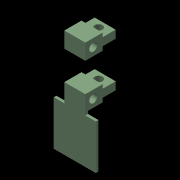
# Autodesk Inventor part: Bearing1
Saved by Autodesk Inventor 2020 (Build 240168000, 168)
## iProperties
Created: 2019-08-05
Part Number: Bearing1
Document SubType Name: Modeling
Designer: Administrator
Density: 1 g/cm^3
Mass: 0.988579 g
Surface Area: 15.6045 cm^2
Volume: 0.988579 cm^3
Material: 一般
Appearance: Green Pastel
Author: Administrator
Autodesk Inventor part; units mm, degrees
ref_plane "YZ Plane" through (0, 0, 0) normal (1, 0, 0) x (0, 1, 0)
ref_plane "XZ Plane" through (0, 0, 0) normal (0, 1, 0) x (-1, 0, 0)
ref_plane "XY Plane" through (0, 0, 0) normal (0, 0, 1) x (1, 0, 0)
sketch "Sketch1" plane through (0, 0, 0) normal (0, 0, 1) x (1, 0, 0)
  circle A0 centre (0, 0) radius 1.5
  line L0 (2.5, 2.5) -> (2.5, -2.5)
  line L1 (2.5, -2.5) -> (-2.5, -2.5)
  line L2 (-2.5, -2.5) -> (-2.5, 2.5)
  line L3 (-2.5, 2.5) -> (2.5, 2.5)
  dimension "d0" = 3
  dimension "d1" = 5
  constraints: 8 end point, 1 centre point, 1 coincident, 10 other
  measures "d0" diameter of A0
  measures "d1" distance of L2.end L0.start
extrude "Extrusion1" add sketch "Sketch1" along normal blind 3
pattern_linear "Rectangular Pattern1" count 2 spacing 17 along (0, 0, 1) of "Extrusion1"
sketch "Sketch2" plane through (0, 0, 0) normal (1, 0, 0) x (0, 1, 0)
  line L0 (-2.5, 17) -> (-2.5, 20) projected
  line L1 (-2.5, 0) -> (-2.5, 3) projected
  line L2 (-2.5, 18.5) -> (-6.05, 18.5) construction
  line L3 (-6.05, 18.5) -> (-6.05, 1.5) construction
  line L4 (-6.05, 1.5) -> (-2.5, 1.5) construction
  line L5 (2.5, 3) -> (-2.5, 3) projected
  line L6 (2.5, 17) -> (-2.5, 17) projected
  line L7 (0, 16.4638) -> (0, 3) construction
  circle A0 centre (-6.05, 18.5) radius 1.5
  circle A1 centre (-6.05, 1.5) radius 1.5
  line L8 (-2.5, 20) -> (-2.5, 21.5)
  line L9 (-2.5, 21.5) -> (-9.05, 21.5)
  line L10 (-9.05, 21.5) -> (-9.05, 15.5)
  line L11 (-9.05, 15.5) -> (-2.5, 15.5)
  line L12 (-2.5, 15.5) -> (-2.5, 17)
  line L13 (-6.05, 10) -> (0, 10) construction
  line L14 (-2.5, 3) -> (-2.5, 0)
  line L15 (-2.5, 1.5) -> (-6.05, 1.5) construction
  circle A2 centre (-6.05, 1.5) radius 1.5
  line L16 (-2.5, 0) -> (-2.5, -1.5)
  line L17 (-2.5, -1.5) -> (-9.05, -1.5)
  line L18 (-9.05, -1.5) -> (-9.05, 4.5)
  line L19 (-9.05, 4.5) -> (-2.5, 4.5)
  line L20 (-2.5, 4.5) -> (-2.5, 3)
  line L21 (-2.5, 17) -> (-2.5, 20)
  dimension "d7" = 6.05
  dimension "d8" = 3
  dimension "d9" = 3
  dimension "d10" = 3
  dimension "d11" = 3
  constraints: 36 end point, 5 symmetric about line, 4 midpoint, 4 perpendicular, 3 centre point, 3 coincident, 3 parallel, 2 collinear, 1 equal radius, 1 point on line, 1 other
  measures "d7" distance between parallel lines of L7 L3
  measures "d8" diameter of A0
  measures "d9" distance between parallel lines of L2 L11
  measures "d10" distance between parallel lines of L9 L2
  measures "d11" distance between parallel lines of L10 L3
extrude "Extrusion2" add sketch "Sketch2" along normal mid plane 8
sketch "Sketch4" plane through (4, -9.05, -1.5) normal (0, 0, -1) x (-1, 0, 0)
  line L0 (8, 0) -> (0, 0) projected
  line L1 (8, 0) -> (8, 6.55) projected
  line L2 (0, 0) -> (8, 0)
  line L3 (8, 0) -> (8, 1)
  line L4 (8, 1) -> (0, 1)
  line L5 (0, 1) -> (0, 0)
  line L6 (0, 1) -> (-4, 1)
  line L7 (-4, 1) -> (-4, 0)
  line L8 (-4, 0) -> (0, 0)
  line L9 (0, 0) -> (0, 1)
  line L10 (8, 0) -> (12, 0)
  line L11 (12, 0) -> (12, 1)
  line L12 (12, 1) -> (8, 1)
  line L13 (8, 1) -> (8, 0)
  circle A0 centre (4, 9.05) radius 1.5 projected
  circle A1 centre (4, 9.05) radius 8.05 construction
  dimension "d14" = 1
  dimension "d15" = 16
  dimension "d16" = 16.1
  dimension "d17" = 0
  constraints: 24 end point, 6 parallel, 3 horizontal, 3 perpendicular, 2 equal length, 1 centre point, 1 coincident, 1 point on line, 1 tangent
  measures "d14" distance between parallel lines of L4 L2
  measures "d15" distance from line of L10.end L7
  measures "d16" diameter of A1
  measures "d17" distance between parallel lines of L8 L0
extrude "Extrusion3" add sketch "Sketch4" along normal blind 18 contours L0 L5 L4 L1 | L1 L12 L11 L10 | L8 L7 L6 L5
sketch "Sketch5" plane through (4, -9.05, -1.5) normal (0, 0, 1) x (1, 0, 0)
  line L0 (0, 1) -> (0, 0) projected
  line L1 (4, 0) -> (0, 0) projected
  line L2 (4, 1) -> (4, 0) projected
  line L3 (0, 1) -> (4, 1) projected
  line L4 (-8, 0) -> (-8, 1) projected
  line L5 (-12, 1) -> (-8, 1) projected
  line L6 (-12, 0) -> (-12, 1) projected
  line L7 (-8, 0) -> (-12, 0) projected
extrude "Extrusion4" cut sketch "Sketch5" against normal blind 1
sketch "Sketch6" plane through (-2.5, 2.5, 0) normal (0, 1, 0) x (1, 0, 0)
  line L0 (0, -20) -> (5, -20) projected
  line L1 (5, -17) -> (5, -20) projected
  line L2 (0, -17) -> (5, -17) projected
  line L3 (0, -17) -> (0, -20) projected
  line L4 (6.5, -21.5) -> (6.5, -15.5) projected
  line L5 (-1.5, -15.5) -> (6.5, -15.5) projected
  line L6 (-1.5, -15.5) -> (-1.5, -21.5) projected
  line L7 (-1.5, -21.5) -> (6.5, -21.5) projected
  line L8 (5, -17) -> (5, -20) projected
  line L9 (5, -20) -> (0, -20) projected
  line L10 (0, -17) -> (0, -20) projected
  line L11 (5, -17) -> (0, -17) projected
  line L12 (6.5, -4.5) -> (6.5, 1.5) projected
  line L13 (-1.5, 1.5) -> (6.5, 1.5) projected
  line L14 (-1.5, 1.5) -> (-1.5, -4.5) projected
  line L15 (-1.5, -4.5) -> (6.5, -4.5) projected
  line L16 (5, 0) -> (5, -3) projected
  line L17 (5, -3) -> (0, -3) projected
  line L18 (0, 0) -> (0, -3) projected
  line L19 (5, 0) -> (0, 0) projected
  line L20 (0, -3) -> (-1.5, -3)
  line L21 (0, 0) -> (-1.5, 0)
  line L22 (5, -3) -> (6.5, -3)
  line L23 (5, 0) -> (6.5, 0)
  line L24 (5, -20) -> (6.5, -20)
  line L25 (5, -17) -> (6.5, -17)
  line L26 (0, -17) -> (-1.5, -17)
  line L27 (0, -20) -> (-1.5, -20)
  constraints: 16 end point, 8 point on line, 6 perpendicular, 2 equal length
extrude "Extrusion5" add sketch "Sketch6" against normal up to surface (5 mm away) contours L27 L6 L26 L3 | L1 L25 L4 L24 | L22 L16 L23 L12 | L14 L21 L18 L20
sketch "Sketch7" plane through (4, 2.5, 20) normal (0, 1, 0) x (1, 0, 0)
  line L0 (0, 0) -> (0, 3) projected
  line L1 (-8, 3) -> (-8, 0) projected
  line L2 (-8, 17) -> (0, 17) projected
  line L3 (0, 17) -> (0, 20) projected
  line L4 (0, 20) -> (-8, 20) projected
  line L5 (-8, 20) -> (-8, 17) projected
  line L6 (-8, 18.5) -> (0, 18.5) construction
  line L7 (-8, 1.5) -> (0, 1.5) construction
  line L8 (-4, 18.5) -> (-4, 1.5) construction
  circle A0 centre (-6.5, 18.5) radius 0.5
  line L9 (-4, 10) -> (-9.0757, 10) construction
  line L10 (0, 1.5) -> (-8, 1.5) construction
  circle A1 centre (-1.5, 18.5) radius 0.5
  circle A2 centre (-6.5, 1.5) radius 0.5
  circle A3 centre (-1.5, 1.5) radius 0.5
  dimension "d24" = 1
  dimension "d25" = 2.5
  constraints: 10 end point, 7 midpoint, 5 symmetric about line, 4 centre point, 1 perpendicular, 1 point on line, 3 other
  measures "d24" diameter of A0
  measures "d25" distance from line of A0.centre L8
extrude "Extrusion6" cut sketch "Sketch7" against normal blind 1.5 contours A0 | A1 | A2 | A3
thread "Thread1" size "M1x0.25" class "6H" standard "ANSI Metric M Profile" full length
thread "Thread2" size "M1x0.25" class "6H" standard "ANSI Metric M Profile" full length
thread "Thread3" size "M1x0.25" class "6H" standard "ANSI Metric M Profile" full length
thread "Thread4" size "M1x0.25" class "6H" standard "ANSI Metric M Profile" full length
